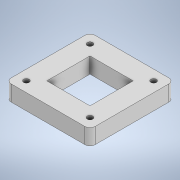
# Autodesk Inventor part: ExtraBase
Saved by Autodesk Inventor 2022 (Build 260153000, 153)
## iProperties
Created: 2022-03-05
Part Number: ExtraBase
Material: Genérico
Document SubType Name: Modeling
Designer: JK
Density: 1 g/cm^3
Appearance: Valor por defecto
Author: JK
Autodesk Inventor part; units mm, degrees
ref_plane "YZ Plane" through (0, 0, 0) normal (1, 0, 0) x (0, 1, 0)
ref_plane "XZ Plane" through (0, 0, 0) normal (0, 1, 0) x (-1, 0, 0)
ref_plane "XY Plane" through (0, 0, 0) normal (0, 0, 1) x (1, 0, 0)
sketch "Boceto1" plane through (0, 0, 0) normal (0, 1, 0) x (-1, 0, 0)
  line L0 (-41.2, 41.2) -> (41.2, 41.2)
  line L1 (41.2, 41.2) -> (41.2, -41.2)
  line L2 (41.2, -41.2) -> (-41.2, -41.2)
  line L3 (-41.2, -41.2) -> (-41.2, 41.2)
  line L4 (-41.2, 41.2) -> (41.2, -41.2) construction
  line L5 (41.2, 41.2) -> (-41.2, -41.2) construction
  line L6 (-21.2, 21.2) -> (21.2, 21.2)
  line L7 (21.2, 21.2) -> (21.2, -21.2)
  line L8 (21.2, -21.2) -> (-21.2, -21.2)
  line L9 (-21.2, -21.2) -> (-21.2, 21.2)
  line L10 (-21.2, 21.2) -> (21.2, -21.2) construction
  line L11 (21.2, 21.2) -> (-21.2, -21.2) construction
  point P0 (0, 0)
  dimension "d0" = 82.4
  dimension "d1" = 82.4
  dimension "d2" = 42.4
  dimension "d3" = 42.4
  constraints: 24 end point, 4 midpoint, 4 parallel, 2 horizontal, 2 perpendicular
  measures "d0" distance of L0.end L1.end
  measures "d1" distance of L1.end L2.end
  measures "d2" distance of L7.end L8.end
  measures "d3" distance of L6.end L7.end
extrude "Extrusión1" add sketch "Boceto1" along normal blind 15.5
sketch "Boceto2" plane through (0, 15.5, 0) normal (0, 1, 0) x (1, 0, 0)
  circle A0 centre (-31.2, -31.2) radius 2.7
  line L0 (-41.2, 41.2) -> (-41.2, -41.2) projected
  line L1 (-41.2, -41.2) -> (41.2, -41.2) projected
  point P0 (0, 0)
  dimension "d6" = 10
  dimension "d7" = 10
  dimension "d8" = 5.4
  constraints: 1 centre point
  measures "d6" distance from line of L0 A0.centre
  measures "d7" distance from line of L1 A0.centre
  measures "d8" diameter of A0
extrude "Extrusión2" cut sketch "Boceto2" against normal through all
fillet "Empalme1" radius 5 1 edges at (-41.2, 7.75, 41.2)
pattern_circular "Patrón circular1" count 4 over 360 about axis through (0, -10, 0) along (0, 1, 0) of "Extrusión2", "Empalme1"
